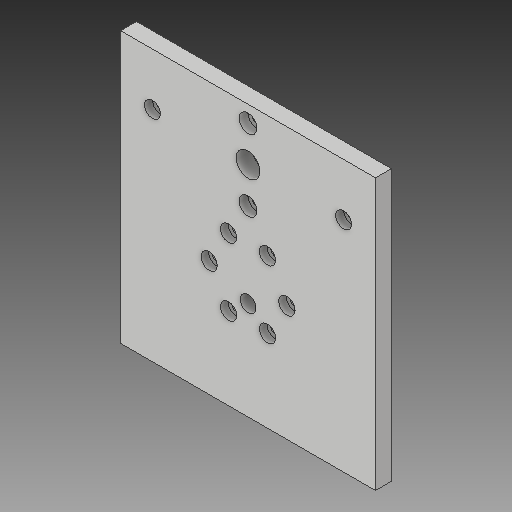
# Autodesk Inventor part: Part3
Saved by Autodesk Inventor 2019 (Build 230136000, 136)
## iProperties
Created: 2018-09-13
Part Number: Part3
Material: Generic
Document SubType Name: Modeling
Designer: drawing
Density: 1 g/cm^3
Appearance: Default
Mass: 67.5939 g
Surface Area: 255.27 cm^2
Volume: 67.5939 cm^3
Author: drawing
Autodesk Inventor part; units mm, degrees
ref_plane "YZ Plane" through (0, 0, 0) normal (1, 0, 0) x (0, 1, 0)
ref_plane "XZ Plane" through (0, 0, 0) normal (0, 1, 0) x (-1, 0, 0)
ref_plane "XY Plane" through (0, 0, 0) normal (0, 0, 1) x (1, 0, 0)
sketch "Sketch1" plane through (0, 0, 0) normal (0, 0, 1) x (1, 0, 0)
  line L0 (0, 0) -> (101.6, 0)
  line L1 (101.6, 0) -> (101.6, 107.95)
  line L2 (101.6, 107.95) -> (0, 107.95)
  line L3 (0, 107.95) -> (0, 0)
  dimension "d0" = 101.6
  dimension "d1" = 107.95
  constraints: 8 end point, 2 parallel, 1 horizontal, 1 perpendicular
  measures "d0" distance of L2.end L1.end
  measures "d1" distance of L1.end L0.end
extrude "Extrusion1" add sketch "Sketch1" along normal blind 6.35
sketch "Sketch2" plane through (0, 0, 6.35) normal (0, 0, 1) x (1, 0, 0)
  line L0 (101.6, 107.95) -> (0, 107.95) projected
  line L1 (101.6, 0) -> (101.6, 107.95) projected
  line L2 (0, 0) -> (101.6, 0) projected
  point P0 (50.8, 87.122)
  point P1 (50.8, 107.95)
  point P2 (101.6, 53.975)
  dimension "d31" = 20.828
  constraints: 2 midpoint, 1 vertical alignment
  measures "d31" distance from line of L0 point (50.8, 87.122)
hole "Hole1" at (50.8, 87.122, 6.35) direction (0, 0, -1) diameter 9.525 depth 19.05 tip angle 118
sketch "Sketch3" plane through (0, 0, 6.35) normal (0, 0, 1) x (1, 0, 0)
  line L0 (101.6, 107.95) -> (0, 107.95) projected
  line L1 (0, 107.95) -> (0, 0) projected
  circle A0 centre (50.8, 87.122) radius 4.7625 projected
  point P0 (12.7, 87.122)
  point P1 (88.9, 87.122)
  dimension "d12" = 12.7
  dimension "d15" = 76.2
  constraints: 2 horizontal alignment
  measures "d12" distance from line of L1 point (12.7, 87.122)
  measures "d15" distance of point (12.7, 87.122) point (88.9, 87.122)
hole "Hole2" at (12.7, 87.122, 6.35) at (88.9, 87.122, 6.35) direction (0, 0, -1) diameter 3.175 depth 19.05 tip angle 118 counterbore diameter 6.35 counterbore depth 3.175
sketch "Sketch4" plane through (0, 0, 6.35) normal (0, 0, 1) x (1, 0, 0)
  circle A0 centre (50.8, 87.122) radius 4.7625 projected
  point P0 (0, 0)
  point P1 (50.8, 39.122)
  dimension "d39" = 48
  constraints: 1 vertical alignment
  measures "d39" distance of A0.centre point (50.8, 39.122)
hole "Hole3" at (50.8, 39.122, 6.35) direction (0, 0, -1) diameter 6.35 depth 19.05 tip angle 118
sketch "Sketch6" plane through (0, 0, 0) normal (0, 0, -1) x (-1, 0, 0)
  circle A0 centre (-50.8, 87.122) radius 4.7625 projected
  point P0 (0, 0)
  point P1 (-50.8, 101.4095)
  point P2 (-50.8, 72.8345)
  dimension "d52" = 28.575
  dimension "d53" = 14.2875
  constraints: 2 vertical alignment
  measures "d52" distance of point (-50.8, 101.41) point (-50.8, 72.835)
  measures "d53" distance of A0.centre point (-50.8, 101.41)
hole "Hole5" at (50.8, 101.4095, 0) at (50.8, 72.8345, 0) direction (0, 0, 1) diameter 3.81 depth 19.05 tip angle 118 counterbore diameter 6.35 counterbore depth 0.508 clearance for "Socket Head Cap Screw" size "#6" standard "Ansi Unified Screw Threads"
sketch "Sketch7" plane through (0, 0, 6.35) normal (0, 0, 1) x (1, 0, 0)
  circle A0 centre (50.8, 101.4095) radius 1.905 projected
  circle A1 centre (50.8, 72.8345) radius 1.905 projected
  point P0 (0, 0)
  constraints: 2 coincident
hole "Hole6" at (50.8, 101.4095, 6.35) at (50.8, 72.8345, 6.35) direction (0, 0, -1) diameter 3.81 depth 19.05 tip angle 118 counterbore diameter 7.1374 counterbore depth 3.5052 clearance for "Socket Head Cap Screw" size "#6" standard "Ansi Unified Screw Threads"
sketch "Sketch8" plane through (0, 0, 6.35) normal (0, 0, 1) x (1, 0, 0)
  circle A0 centre (50.8, 46.122) radius 15.5
  circle A1 centre (50.8, 39.122) radius 3.175 projected
  point P0 (0, 0)
  point P1 (66.3, 46.122)
  point P2 (58.55, 59.5454)
  point P3 (43.05, 59.5454)
  point P4 (35.3, 46.122)
  point P5 (43.05, 32.6986)
  point P6 (58.55, 32.6986)
  dimension "d68" = 31
  dimension "d69" = 7
  dimension "d79" = 360
  constraints: 2 horizontal alignment, 1 vertical alignment, 9 other
  measures "d69" distance of A1.centre point (50.8, 46.122)
hole "Hole8" at (66.3, 46.122, 6.35) at (58.55, 59.5454, 6.35) at (43.05, 59.5454, 6.35) at (35.3, 46.122, 6.35) at (43.05, 32.6986, 6.35) at (58.55, 32.6986, 6.35) direction (0, 0, -1) diameter 3.4036 depth 12.2936 tip angle 118 counterbore diameter 6.5024 counterbore depth 2.9972 clearance for "Socket Head Cap Screw" size "M3" standard "Ansi Metric M Profile"
equation "\"d53\" = 0.5 * d52"
body "Solid1"
